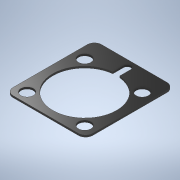
# Autodesk Inventor part: cylinder head gasket
Saved by Autodesk Inventor 2020 (Build 240168000, 168)
## iProperties
Created: 2020-08-05
Part Number: cylinder head gasket
Material: Generic
Document SubType Name: Modeling
Designer: benny
Density: 1 g/cm^3
Appearance: Glossy - Black
Author: benny
Autodesk Inventor part; units mm, degrees
ref_plane "YZ Plane" through (0, 0, 0) normal (1, 0, 0) x (0, 1, 0)
ref_plane "XZ Plane" through (0, 0, 0) normal (0, 1, 0) x (-1, 0, 0)
ref_plane "XY Plane" through (0, 0, 0) normal (0, 0, 1) x (1, 0, 0)
sketch "Sketch1" plane through (0, 0, 0) normal (0, 1, 0) x (-1, 0, 0)
  line L0 (-22.5, 22) -> (22.5, 22)
  line L1 (22.5, 22) -> (22.5, -28)
  line L2 (22.5, -28) -> (-22.5, -28)
  line L3 (-22.5, -28) -> (-22.5, 22)
  line L4 (-22.5, 22) -> (22.5, -28) construction
  line L5 (22.5, 22) -> (-22.5, -28) construction
  point P0 (0, 0)
  point P1 (0, -3)
  dimension "d0" = 45
  dimension "d1" = 50
  dimension "d26" = 22
  dimension "d35" = 3
  constraints: 12 end point, 2 midpoint, 2 parallel, 1 horizontal, 1 perpendicular
  measures "d0" distance of L1.end L2.end
  measures "d1" distance of L0.end L1.end
  measures "d26" distance from line of L0 point (0, 0)
  measures "d35" distance of point (0, 0) point (0, -3)
extrude "Extrusion1" add sketch "Sketch1" along normal blind 1
fillet "Fillet1" radius 4 4 edges at (22.5, 0.5, 22) (-22.5, 0.5, 22) (-22.5, 0.5, -28) (22.5, 0.5, -28)
sketch "Sketch2" plane through (0, 1, 0) normal (0, 1, 0) x (1, 0, 0)
  circle A0 centre (0, 0) radius 18
  dimension "d5" = 36
  constraints: 2 coincident, 1 centre point
  measures "d5" diameter of A0
extrude "Extrusion2" cut sketch "Sketch2" against normal blind 1
sketch "Sketch4" plane through (0, 1, 0) normal (0, 1, 0) x (1, 0, 0)
  line L0 (0, 0) -> (0, 24)
  circle A0 centre (0, 24) radius 2
  dimension "d15" = 24
  dimension "d16" = 4
  constraints: 2 end point, 1 centre point, 1 coincident, 1 vertical
  measures "d15" distance of L0.start L0.end
  measures "d16" diameter of A0
extrude "Extrusion4" cut sketch "Sketch4" against normal blind 1
sketch "Sketch6" plane through (0, 1, 0) normal (0, 1, 0) x (1, 0, 0)
  line L0 (0, 0) -> (-16.2635, -16.2635)
  line L1 (0, 0) -> (23, 0) construction
  circle A0 centre (-16.2635, -16.2635) radius 3.5
  dimension "d27" = 23
  dimension "d28" = 135
  dimension "d29" = 7
  constraints: 4 end point, 1 centre point, 1 coincident, 1 equal length, 1 horizontal
  measures "d27" distance of L0.start L0.end
  measures "d28" angle of L0 L1
  measures "d29" diameter of A0
extrude "Extrusion6" cut sketch "Sketch6" against normal blind 1
pattern_circular "Circular Pattern2" count 4 over 360 about axis through (0, 1, 0) along (0, -1, 0) of "Extrusion6"
sketch "Sketch7" plane through (0, 1, 0) normal (0, 1, 0) x (1, 0, 0)
  circle A0 centre (0, 24) radius 2 projected
  line L0 (-2, 24) -> (2, 24)
  line L1 (2, 24) -> (2, 16.9312)
  line L2 (2, 16.9312) -> (-2, 16.9312)
  line L3 (-2, 16.9312) -> (-2, 24)
  point P0 (0, 0)
  constraints: 8 end point, 2 parallel, 2 point on circle, 1 horizontal, 1 perpendicular
extrude "Extrusion7" cut sketch "Sketch7" against normal blind 1 contours L1 L2 L3 A0
body "Solid1"
